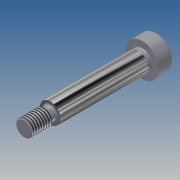
# Autodesk Inventor part: SCREW, SHOULDER, P, 12
Saved by Autodesk Inventor 2022.4 (Build 264492000, 492)
## iProperties
Company: Cooper Bussmann Denmark
Category: _
Manager: 607-50165
Created: 2001-02-28
Part Number: SCREW, SHOULDER, P, 12
Document SubType Name: Modeling
Designer: Peter Damgaard
Material: Steel, High Strength Low Alloy
Density: 7.84 g/cm^3
Appearance: Metal-Steel(Polish)
Checked By: 0001004421
User Status: Released
Description: SCREW, SHOULDER, P, 12.9, 10X45
Engr Approved By: P
Mfg Approved By: -
Mass: 42.8389 g
Surface Area: 25.7748 cm^2
Volume: 5.46414 cm^3
Control State: 0
Master: False
Checked Out: False
Shininess: 60.0
PTC_WM_ITERATION: 2
PTC_WM_ORGANIZATION_ID: CLWC
PTC_WM_LIFECYCLE: CLWC_CAD_LC
THIRD_DESCRIPTION: -
FIRST_DESCRIPTION: -
SECOND_DESCRIPTION: -
CN_SERVICEABLE: _
CN_MASS: 0.042839
CL_runCount: 1
FinishProperty: ToBeSet
Density: 7.84
Volumn: 1.0724371659246204
Area: 8.535162991116971
PropertySet Name: Model Information
Author: -
Revision Number: A
Subject: _
Keywords: -
Autodesk Inventor part; units mm, degrees
ref_plane "YZ Plane" through (0, 0, 0) normal (1, 0, 0) x (0, 1, 0)
ref_plane "XZ Plane" through (0, 0, 0) normal (0, 1, 0) x (-1, 0, 0)
ref_plane "XY Plane" through (0, 0, 0) normal (0, 0, 1) x (1, 0, 0)
sketch "Sketch1" plane through (0, 0, 0) normal (0, 0, 1) x (1, 0, 0)
  line L0 (0, 0) -> (-5, 0)
  line L1 (-5, 0) -> (-5, -43.15)
  line L2 (-5, -43.15) -> (0, -43.15)
  line L3 (0, -43.15) -> (0, 0)
  line L4 (0, 0) -> (-13.1356, 0) construction
  dimension "d1" = 43.15
  dimension "d2" = 5
  constraints: 10 end point, 2 parallel, 1 horizontal, 1 perpendicular, 1 point on line
  measures "d1" distance of L0.end L1.end
  measures "d2" distance of L0.start L0.end
revolve "Shoulder" add sketch "Sketch1" angle 360 about axis through (0, -43.15, 0) along (0, 1, 0)
sketch "Sketch2" plane through (0, 0, 0) normal (0, 1, 0) x (1, 0, 0)
  circle A0 centre (0, 0) radius 5 projected
  circle A1 centre (0, 0) radius 4.76
  dimension "d3" = 9.52
  constraints: 1 centre point, 1 concentric
  measures "d3" diameter of A1
extrude "Shoulder_neck" add sketch "Sketch2" along normal blind 1.85 contours A1
sketch "Sketch3" plane through (0, 1.85, 0) normal (0, 1, 0) x (1, 0, 0)
  circle A0 centre (0, 0) radius 4.76 projected
  circle A1 centre (0, 0) radius 8.1
  dimension "d6" = 16.2
  constraints: 1 centre point, 1 concentric
  measures "d6" diameter of A1
extrude "Head" add sketch "Sketch3" along normal blind 7 contours A0 | A1
sketch "Sketch4" plane through (0, -43.15, 0) normal (0, -1, 0) x (1, 0, 0)
  circle A0 centre (0, 0) radius 5 projected
  circle A1 centre (0, 0) radius 3.09
  dimension "d9" = 6.18
  constraints: 1 centre point, 1 concentric
  measures "d9" diameter of A1
extrude "Thread_neck" add sketch "Sketch4" along normal blind 2.6 contours A1
sketch "Sketch5" plane through (0, -45.75, 0) normal (0, -1, 0) x (1, 0, 0)
  circle A0 centre (0, 0) radius 3.09 projected
  circle A1 centre (0, 0) radius 4
  dimension "d12" = 8
  constraints: 1 centre point, 1 concentric
  measures "d12" diameter of A1
extrude "Thread_shoulder" add sketch "Sketch5" along normal blind 10.4 contours A0 | A1
sketch "Sketch6" plane through (0, 8.85, 0) normal (0, 1, 0) x (1, 0, 0)
  circle A0 centre (0, 0) radius 8.1 projected
  circle A1 centre (0, 0) radius 2.5 construction
  line L0 (-2.5, 1.4434) -> (-2.5, -1.4434)
  line L1 (-2.5, -1.4434) -> (0, -2.8868)
  line L2 (0, -2.8868) -> (2.5, -1.4434)
  line L3 (2.5, -1.4434) -> (2.5, 1.4434)
  line L4 (2.5, 1.4434) -> (0, 2.8868)
  line L5 (0, 2.8868) -> (-2.5, 1.4434)
  dimension "d15" = 5
  constraints: 12 end point, 6 equal length, 6 tangent, 1 centre point, 1 concentric, 1 parallel, 1 vertical
  measures "d15" diameter of A1
extrude "Hex" cut sketch "Sketch6" against normal blind 4.2 contours L5 L4 L3 L2 L1 L0
chamfer "Chamfer1" distance 0.24 angle 30 1 edges at (5, 0, 0) measured on face at (-4.8255, 0, -0.7786)
fillet "Fillet1" radius 0.4 1 edges at (-4.76, 1.85, 0)
chamfer "Chamfer2" distance 0.5 angle 30 1 edges at (-8.1, 8.85, 0) measured on face at (7.9951, 6.5167, 1.2993)
chamfer "Chamfer3" distance 0.625 angle 30 1 edges at (-4, -56.15, 0) measured on face at (0.7574, -56.15, 1.0973)
fillet "Fillet2" radius 0.7 1 edges at (-3.09, -43.15, 0)
chamfer "Chamfer7" distance 0.91 angle 30 1 edges at (-4, -45.75, 0) measured on face at (3.6579, -45.75, -0.3191)
thread "Thread" size "M8x1.25" class "6g" standard "ANSI Metric M Profile" full length
equation "\"d3\" = Shoulder_neck_dia"
equation "\"d4\" = Shoulder_neck_length"
equation "\"d6\" = Head_diameter"
equation "\"d7\" = Head_height"
equation "\"d9\" = Thread_neck_dia"
equation "\"d10\" = Thread_neck_length"
equation "\"d12\" = Thread_diameter"
equation "\"d13\" = Thread_length - Thread_neck_length"
equation "\"d15\" = Hex_size"
equation "\"d16\" = Hex_length"
equation "\"d18\" = -0.5 * Shoulder_neck_dia + 0.5 * Shoulder_diameter"
equation "\"d64\" = -0.5 * Shoulder_neck_dia + 0.5 * Shoulder_diameter"
equation "\"d21\" = 0.1 * Hex_size"
equation "\"d65\" = 0.1 * Hex_size"
equation "\"d23\" = 0.5 * Thread_pitch"
equation "\"d66\" = 0.5 * Thread_pitch"
equation "\"d25\" = Thread_neck_radius"
equation "\"d60\" = -0.5 * Thread_neck_dia + 0.5 * Thread_diameter"
equation "\"d67\" = -0.5 * Thread_neck_dia + 0.5 * Thread_diameter"
equation "\"d1\" = Shoulder_length - Shoulder_neck_length"
equation "\"d2\" = 0.5 * Shoulder_diameter"
equation "\"Shoulder_length\" = 45"
equation "\"Shoulder_neck_dia\" = 9.52"
equation "\"Thread_diameter\" = 8"
equation "\"Thread_length\" = 13"
equation "\"Head_diameter\" = 16.2"
equation "\"Head_height\" = 7"
equation "\"Thread_neck_dia\" = 6.18"
equation "\"Hex_size\" = 5"
equation "\"Hex_length\" = 4.2"
equation "\"Thread_pitch\" = 1.25"
equation "\"Shoulder_neck_length\" = 1.85"
equation "\"Thread_neck_length\" = 2.6"
equation "\"Thread_neck_radius\" = 0.7"
equation "\"Shoulder_diameter\" = 10"
body "Solid1"
